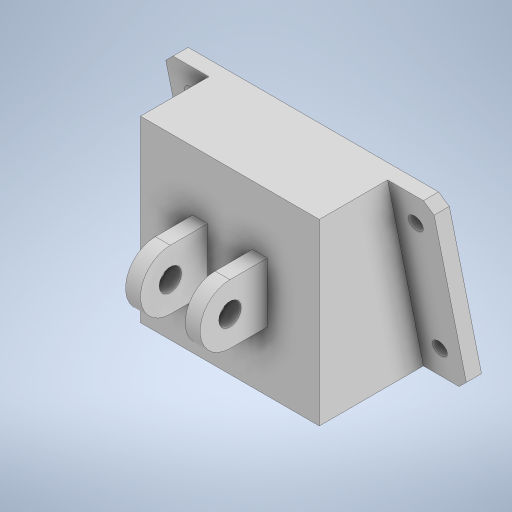
# Autodesk Inventor part: Base
Saved by Autodesk Inventor 2024 (Build 280153000, 153)
## iProperties
Created: 2023-06-06
Part Number: Base
Material: Generic
Document SubType Name: Modeling
Designer: Samyak Gosalia
Density: 1 g/cm^3
Appearance: Default
Author: Samyak Gosalia
Autodesk Inventor part; units mm, degrees
ref_plane "XZ Plane" through (0, 0, 0) normal (0, 1, 0) x (-1, 0, 0)
ref_plane "XY Plane" through (0, 0, 0) normal (0, 0, 1) x (1, 0, 0)
ref_plane "Work Plane1" through (30, 0, 0) normal (1, 0, 0) x (0, 1, 0)
sketch "Sketch1" plane through (0, 0, 0) normal (0, 0, 1) x (1, 0, 0)
  line L0 (0, 0) -> (60, 0)
  line L1 (60, 0) -> (60, 60)
  line L2 (60, 60) -> (0, 60)
  line L3 (0, 60) -> (0, 0)
  dimension "d0" = 60
  dimension "d1" = 60
  constraints: 8 end point, 2 parallel, 1 horizontal, 1 perpendicular
  measures "d0" distance of L2.end L1.end
  measures "d1" distance of L1.end L0.end
extrude "Extrusion1" add sketch "Sketch1" along normal blind 40
sketch "Sketch3" plane through (60, 0, 0) normal (1, 0, 0) x (0, 0, -1)
  line L0 (0, 0) -> (-12.0001, 60)
  line L1 (0, 60) -> (-40, 60) projected
  line L2 (0, 0) -> (61.1882, 0) construction
  arc A0 (0, 60) -> (-12.0001, 60) centre (-6, 30) ccw
  line L3 (0, 0) -> (0, 60) projected
  line L4 (0, 60) -> (0, 0)
  dimension "d7" = 101.31
  constraints: 6 end point, 2 point on circle, 1 centre point, 1 collinear, 1 equal length, 1 horizontal, 1 midpoint, 1 point on line
  measures "d7" angle of L2 L0
extrude "Extrusion3" cut sketch "Sketch3" against normal through all contours L0 L1 L3
sketch "Sketch4" plane through (0, 0, 40) normal (0, 0, 1) x (1, 0, 0)
  line L0 (0, 0) -> (60, 0) construction
  line L1 (30, 0) -> (30, 60) construction
  line L2 (60, 60) -> (0, 60) construction
  line L3 (0, 60) -> (0, 0) construction
  line L4 (0, 30) -> (60, 30) construction
  line L5 (60, 0) -> (60, 60) construction
  line L6 (22.5, 20) -> (22.5, 40)
  line L7 (37.5, 20) -> (37.5, 40)
  line L8 (17.5, 20) -> (17.5, 40)
  line L9 (42.5, 20) -> (42.5, 40)
  line L10 (17.5, 20) -> (22.5, 20)
  line L11 (37.5, 20) -> (42.5, 20)
  line L12 (17.5, 40) -> (22.5, 40)
  line L13 (37.5, 40) -> (42.5, 40)
  dimension "d12" = 7.5
  dimension "d13" = 7.5
  dimension "d14" = 5
  dimension "d15" = 20
  dimension "d16" = 5
  dimension "d17" = 20
  dimension "d18" = 20
  dimension "d19" = 20
  constraints: 20 end point, 7 perpendicular, 4 midpoint, 1 parallel
  measures "d12" distance between parallel lines of L6 L1
  measures "d13" distance between parallel lines of L1 L7
  measures "d14" distance of L7.end L9.end
  measures "d15" distance of L9.start L9.end
  measures "d16" distance of L8.end L6.end
  measures "d17" distance of L8.start L8.end
  measures "d18" distance between parallel lines of L0 L10
  measures "d19" distance between parallel lines of L0 L11
extrude "Extrusion4" add sketch "Sketch4" along normal blind 22.5
fillet "Fillet1" radius 10 4 edges at (20, 20, 62.5) (20, 40, 62.5) (40, 20, 62.5) (40, 40, 62.5)
sketch "Sketch5" plane through (42.5, 20, 40) normal (1, 0, 0) x (0, 0, -1)
  arc A0 (-12.5, 20) -> (-12.5, 0) centre (-12.5, 10) ccw projected
  line L0 (-12.5, 0) -> (-12.5, 20) construction
  circle A1 centre (-12.5, 10) radius 3.75
  point P0 (40, -20)
  dimension "d23" = 7.5
  constraints: 2 end point, 1 centre point, 1 coincident, 1 vertical
  measures "d23" diameter of A1
extrude "Extrusion5" cut sketch "Sketch5" against normal through all
sketch "Sketch6" plane through (30, 0, 0) normal (1, 0, 0) x (0, 1, 0)
  line L0 (60, 12.0001) -> (60, 40) projected
  line L1 (0, 0) -> (60, 12.0001)
  line L2 (60, 12.0001) -> (60, 17.0991)
  line L3 (60, 17.0991) -> (0, 5.099)
  line L4 (0, 5.099) -> (0, 0)
  dimension "d27" = 5
  constraints: 8 end point, 2 parallel, 1 point on line
  measures "d27" distance between parallel lines of L1 L3
extrude "Extrusion6" add sketch "Sketch6" along normal mid plane 90
sketch "Sketch7" plane through (60, 0, 5.099) normal (0, -0.1961173, 0.9805804) x (1, 0, 0)
  circle A0 centre (7.5, 10) radius 2.5
  circle A1 centre (7.5, 51.1882) radius 2.5
  line L0 (15, 61.1882) -> (15, 0) projected
  line L1 (0, 0) -> (15, 0) projected
  line L2 (0, 61.1882) -> (15, 61.1882) projected
  point P0 (-60, -1)
  dimension "d30" = 5
  dimension "d31" = 5
  dimension "d32" = 7.5
  dimension "d33" = 7.5
  dimension "d34" = 10
  dimension "d35" = 10
  constraints: 2 centre point
  measures "d30" diameter of A0
  measures "d31" diameter of A1
  measures "d32" distance from line of L0 A0.centre
  measures "d33" distance from line of L0 A1.centre
  measures "d34" distance from line of L1 A0.centre
  measures "d35" distance from line of L2 A1.centre
extrude "Extrusion7" cut sketch "Sketch7" against normal through all
mirror "Mirror1" about plane through (30, 0, 0) normal (1, 0, 0) of "Extrusion7"
chamfer "Chamfer1" distance 3 angle 45 4 edges at (75, 0, 2.5495) (75, 60, 14.5496) (-15, 0, 2.5495) (-15, 60, 14.5496)
body "Solid1"
